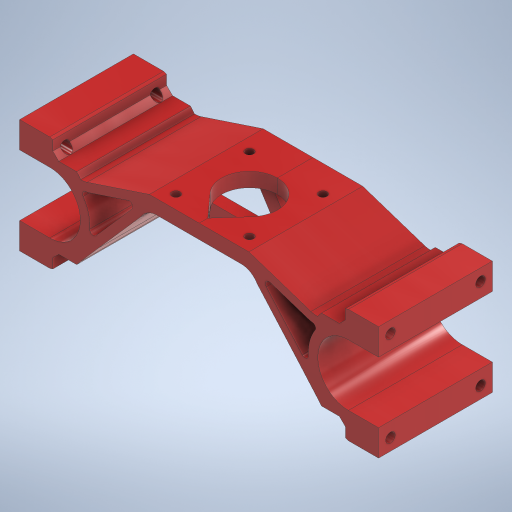
# Autodesk Inventor part: XZ_Main
Saved by Autodesk Inventor 2023 (Build 270158000, 158)
## iProperties
Created: 2023-11-25
Part Number: XZ_Main
Material: Generic
Document SubType Name: Modeling
Designer: danie
Density: 1 g/cm^3
Appearance: Default
Author: danie
Autodesk Inventor part; units mm, degrees
ref_plane "YZ Plane" through (0, 0, 0) normal (1, 0, 0) x (0, 1, 0)
ref_plane "XZ Plane" through (0, 0, 0) normal (0, 1, 0) x (-1, 0, 0)
ref_plane "XY Plane" through (0, 0, 0) normal (0, 0, 1) x (1, 0, 0)
sketch "Sketch1" plane through (0, 0, 0) normal (0, 0, 1) x (1, 0, 0)
  line L0 (102.5, 88.05) -> (102.5, 93.9228)
  line L1 (124.5356, 116.5109) -> (111.3979, 95.8971)
  arc A0 (111.3979, 95.8971) -> (112.6628, 93.591) centre (112.6628, 95.091) ccw
  line L2 (112.6628, 93.591) -> (143.9197, 93.591)
  arc A1 (143.9197, 93.591) -> (145.0463, 96.0813) centre (143.9197, 95.091) ccw
  line L3 (145.0463, 96.0813) -> (126.9272, 116.695)
  arc A2 (126.9272, 116.695) -> (124.5356, 116.5109) centre (125.8005, 115.7047) ccw
  line L4 (102.5, 120.5) -> (117.1944, 120.5)
  arc A3 (118.4593, 118.1938) -> (117.1944, 120.5) centre (117.1944, 119) ccw
  line L5 (118.4593, 118.1938) -> (103.7515, 95.1166)
  arc A4 (102.4866, 94.4228) -> (103.7515, 95.1166) centre (102.4866, 95.9228) ccw
  line L6 (102.5, 120.5) -> (102.5, 126)
  line L7 (102.5, 94.4229) -> (102.5, 120.5)
  line L8 (102.5, 93.9228) -> (102.5, 94.4229)
  arc A5 (165.5, 126.5) -> (164.2, 126.082) centre (172.5, 102.5) ccw
  line L9 (178.2, 126.5) -> (178.2, 115.4)
  line L10 (178.2, 115.4) -> (165.5, 115.4)
  arc A6 (165.5, 115.4) -> (165.5, 89.6) centre (165.5, 102.5) ccw
  line L11 (165.5, 89.6) -> (178.2, 89.6)
  line L12 (178.2, 89.6) -> (178.2, 78.5)
  line L13 (165.5, 78.5) -> (178.2, 78.5)
  line L14 (165.5, 126.5) -> (178.2, 126.5)
  arc A7 (151.3929, 111.8134) -> (150.368, 114.1215) centre (150.1404, 112.6388) ccw
  arc A8 (148.2227, 114.6331) -> (150.368, 114.1215) centre (152.4166, 127.4653) ccw
  line L15 (148.2227, 114.6331) -> (132.4493, 119.8522)
  arc A9 (132.4493, 119.8522) -> (130.8515, 117.4378) centre (131.9781, 118.4281) ccw
  line L16 (130.8515, 117.4378) -> (146.0215, 100.1793)
  arc A10 (146.0215, 100.1793) -> (148.6442, 101.2779) centre (147.1482, 101.1696) ccw
  line L17 (102.5, 88.05) -> (102.5, 87.55)
  line L18 (102.5, 87.55) -> (152.4626, 87.55)
  line L19 (102.5, 126) -> (102.5, 126.5)
  line L20 (164.2, 126.082) -> (164.2, 125.5997)
  line L21 (164.2, 125.5997) -> (152.4626, 125.5997)
  line L22 (152.4626, 125.5997) -> (145.8246, 126.5)
  line L23 (145.8246, 126.5) -> (102.5, 126.5)
  arc A11 (151.3929, 111.8134) -> (148.6442, 101.2779) centre (165.6017, 102.4801) ccw
  line L24 (145.0463, 96.0813) -> (152.4626, 87.55)
  line L25 (117.1944, 120.5) -> (119.9291, 120.5)
  arc A12 (126.9272, 116.695) -> (119.9291, 120.5) centre (120.2433, 112.74) ccw
  line L26 (149.6996, 117.831) -> (123.5, 126.5) projected
  line L27 (164.2, 125.5997) -> (164.2, 121.975)
  line L28 (164.2, 121.975) -> (161.7, 119.475)
  line L29 (161.7, 119.475) -> (154.1465, 119.475)
  arc A13 (149.6996, 117.831) -> (152.4626, 117.45) centre (152.1133, 125.1257) ccw
  line L30 (164.2, 78.918) -> (164.2, 83.025)
  line L31 (164.2, 83.025) -> (161.7, 85.525)
  line L32 (161.7, 85.525) -> (154.1465, 85.525)
  arc A14 (164.2, 78.918) -> (165.5, 78.5) centre (172.5, 102.5) ccw
  arc A15 (164.2, 126.082) -> (154.1465, 119.475) centre (172.5, 102.5) ccw
  arc A16 (154.1465, 119.475) -> (154.1465, 85.525) centre (172.5, 102.5) ccw
  point P0 (0, 0)
  point P1 (177.7, 79)
  point P2 (177.7, 89.1)
  point P3 (165.5, 89.1)
  point P4 (165.5, 115.9)
  point P5 (177.7, 115.9)
  point P6 (177.7, 126)
  point P7 (164.2, 126)
  point P8 (145.0571, 96.0688)
  point P9 (162.9396, 125.5997)
  point P10 (154.1465, 85.525)
  point P11 (152.4626, 117.45)
  dimension "d10" = 25
  dimension "d14" = 0.5
  dimension "d15" = 17
  constraints: 64 end point, 41 point on circle, 17 centre point, 4 perpendicular, 4 point on line, 4 vertical, 1 parallel, 1 tangent
  measures "d10" radius of A5
  measures "d14" distance of L0.start L17.end
  measures "d15" radius of A11
extrude "Extrusion1" add sketch "Sketch1" along normal blind 48 contours A16 A10 A11 A7 L29 L28 L27 L20 A5 L14 L9 L10 A6 L11 L12 L13 A14 L30 L31 L32 | L24 L3 A12 L25 L4 L6 L19 L23 L26 A13 A16 A8 L15 A9 L16 A10
extrude "Extrusion2" add sketch "Sketch1" along normal blind 5 contours L0 L8 A4 L5 A3 L25 A12 A2 L1 A0 L2 A1 L24 L18 L17
sketch "Sketch2" plane through (102.5, 120.5, 48) normal (0, -1, 0) x (1, 0, 0)
  line L0 (0, -48) -> (14.6944, -48) projected
  line L1 (0, 0) -> (17.4291, 0) projected
  line L2 (0, -48) -> (0, 0) projected
  line L3 (0, -48) -> (49.9626, -48) projected
  line L4 (49.9626, -48) -> (49.9626, -43) projected
  line L5 (0, -43) -> (49.9626, -43) projected
  line L6 (0, -48) -> (0, -43) projected
  line L7 (15.5, -36.7512) -> (-15.5, -36.7512)
  line L8 (-15.5, -36.7512) -> (-15.5, -5.7512)
  line L9 (-15.5, -5.7512) -> (0, -5.7512)
  line L10 (15.5, -5.7512) -> (15.5, -36.7512)
  line L11 (15.5, -36.7512) -> (-15.5, -5.7512) construction
  line L12 (-15.5, -36.7512) -> (15.5, -5.7512) construction
  arc A0 (8.3071, -29.5583) -> (8.3065, -12.9447) centre (-0.0007, -21.2518) ccw
  line L13 (0, -3.6899) -> (8.318, -12.9332)
  arc A1 (0, -32.9999) -> (8.3071, -29.5583) centre (-0.0007, -21.2518) ccw
  arc A2 (8.3065, -12.9447) -> (0, -32.9999) centre (-0.0007, -21.2518) ccw
  line L14 (8.318, -12.9332) -> (8.732, -13.3933)
  line L15 (1.855, -5.7512) -> (15.5, -5.7512)
  line L16 (0, -5.7512) -> (1.855, -5.7512)
  line L17 (0, -3.6899) -> (0, -5.7512)
  line L18 (17.4291, -43) -> (17.4291, 0) projected
  line L19 (14.6944, -43) -> (14.6944, -48) projected
  line L20 (14.6944, -43) -> (17.4291, -43) projected
  point P0 (-102.5, -48)
  point P1 (0, -21.2512)
  point P2 (15.5, -36.7512)
  dimension "d21" = 31
  dimension "d22" = 31
  constraints: 22 end point, 8 point on circle, 6 point on line, 4 parallel, 4 tangent, 3 centre point, 3 coincident, 2 midpoint, 1 collinear, 1 horizontal, 1 perpendicular
  measures "d21" distance of L8.end L10.start
  measures "d22" distance of L7.end L8.end
extrude "Extrusion3" cut sketch "Sketch2" against normal through all contours L2 A2 A0 A1 | L2 L16 L13 L14 A0 A2 | L2 L13 L16
hole "Hole1" at (118, 120.5, 42.2488) at (118, 120.5, 11.2488) direction (0, 1, 0) diameter 3.4 end through all clearance for "Countersunk Flat Head Screw ISO 2009/7046" size "M3" standard "ISO"
sketch "Sketch4" plane through (178.2, 78.5, 0) normal (1, 0, 0) x (0, 0, -1)
  line L0 (0, 0) -> (0, 11.1) projected
  line L1 (0, 11.1) -> (-48, 11.1) projected
  line L2 (-48, 0) -> (-48, 11.1) projected
  line L3 (0, 0) -> (-48, 0) projected
  line L4 (0, 36.9) -> (0, 48) projected
  line L5 (0, 48) -> (-48, 48) projected
  line L6 (-48, 36.9) -> (-48, 48) projected
  line L7 (0, 36.9) -> (-48, 36.9) projected
  line L8 (-44.3101, 48) -> (-48, 48) projected
  line L9 (0, 0) -> (-48, 48)
  line L10 (-48, 0.418) -> (-48, 0) projected
  line L11 (0, 48) -> (0, 42) projected
  line L12 (-48, 0) -> (0, 48)
  line L13 (-5, 5) -> (-43, 5)
  line L14 (-43, 5) -> (-43, 43)
  line L15 (-43, 43) -> (-5, 43)
  line L16 (-5, 43) -> (-5, 5)
  line L17 (-5, 5) -> (-43, 43) construction
  line L18 (-43, 5) -> (-5, 43) construction
  point P0 (0, -78.5)
  point P1 (-24, 24)
  dimension "d33" = 38
  dimension "d34" = 38
  constraints: 16 end point, 4 coincident, 3 midpoint, 2 parallel, 1 horizontal, 1 perpendicular
  measures "d33" distance of L14.end L15.end
  measures "d34" distance of L13.end L14.end
hole "Hole2" at (178.2, 121.5, 5) at (178.2, 121.5, 43) at (178.2, 83.5, 43) at (178.2, 83.5, 5) direction (-1, 0, 0) diameter 4 depth 18
sketch "Sketch5" plane through (178.2, 78.5, 0) normal (1, 0, 0) x (0, 0, -1)
  circle A0 centre (-43, 5) radius 2 projected
  circle A1 centre (-5, 5) radius 2 projected
  line L0 (0, 0) -> (0, 11.1) projected
  line L1 (0, 11.1) -> (-48, 11.1) projected
  line L2 (-48, 0) -> (-48, 11.1) projected
  line L3 (0, 0) -> (-48, 0) projected
  circle A2 centre (-5, 43) radius 2 projected
  circle A3 centre (-43, 43) radius 2 projected
  line L4 (0, 36.9) -> (0, 48) projected
  line L5 (0, 48) -> (-48, 48) projected
  line L6 (-48, 36.9) -> (-48, 48) projected
  line L7 (0, 36.9) -> (-48, 36.9) projected
  line L8 (-48, 39.331) -> (-48, 48) projected
  line L9 (0, 0) -> (-48, 48)
  line L10 (0, 48) -> (-15.0001, 48) projected
  line L11 (-48, 0) -> (0, 48)
  point P0 (0, -78.5)
  point P1 (-24, 24)
  constraints: 4 end point, 1 midpoint
mirror "Mirror1" about plane through (102.5, 94.4229, 0) normal (-1, 0, 0)
sketch "Sketch6" plane through (26.8, 78.5001, 0) normal (-1, 0, 0) x (0, 0, 1)
  circle A0 centre (43, 5) radius 2 projected
  circle A1 centre (5, 5) radius 2 projected
  line L0 (0, 0) -> (0, 11.1) projected
  line L1 (0, 0) -> (48, 0) projected
  line L2 (48, 0) -> (48, 11.1) projected
  line L3 (0, 11.1) -> (48, 11.1) projected
  circle A2 centre (5, 43) radius 2 projected
  circle A3 centre (43, 43) radius 2 projected
  line L4 (0, 36.9) -> (0, 48) projected
  line L5 (0, 36.9) -> (48, 36.9) projected
  line L6 (48, 36.9) -> (48, 48) projected
  line L7 (0, 48) -> (48, 48) projected
  line L8 (48, 0.0001) -> (48, 11.1001) projected
  line L9 (0, 48) -> (0, 48) projected
  line L10 (48, 0.0001) -> (0, 48)
  line L11 (0, 48) -> (48, 48) projected
  line L12 (0, 0) -> (48, 48)
  point P0 (0, -78.5001)
  point P1 (24, 24)
  constraints: 4 end point, 1 midpoint
body "Solid1"
